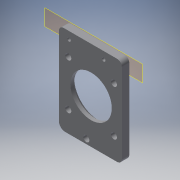
# Autodesk Inventor part: cellSTORM_inverted_chiptray_v0
Saved by Autodesk Inventor 2019.4 (Build 234330000, 330)
## iProperties
Created: 2020-11-09
Part Number: cellSTORM_inverted_chiptray_v0
Material: Generic
Document SubType Name: Modeling
Designer: diederichbenedict
Density: 1 g/cm^3
Appearance: Default
Author: diederichbenedict
Autodesk Inventor part; units mm, degrees
ref_plane "YZ Plane" through (0, 0, 0) normal (1, 0, 0) x (0, 1, 0)
ref_plane "XZ Plane" through (0, 0, 0) normal (0, 1, 0) x (-1, 0, 0)
ref_plane "XY Plane" through (0, 0, 0) normal (0, 0, 1) x (1, 0, 0)
ref_plane "Work Plane1" through (0, 0, 0) normal (0, 0, 1) x (1, 0, 0)
sketch "Sketch1" plane through (0, 0, 0) normal (0, 0, 1) x (1, 0, 0)
  line L0 (10.8382, -62.5107) -> (10.8382, 0.6668)
  line L1 (6.9805, -66.3684) -> (-18, -66.3684)
  line L2 (10.8382, -5.7047) -> (9.6808, -5.7047) construction
  line L3 (10.8382, 0.6668) -> (10.8382, 2.1422)
  line L4 (-40.1739, 0.853) -> (-40.1739, 2.1422)
  line L5 (6.9805, 6) -> (-36.3161, 6)
  circle A0 centre (-3.9646, 0) radius 1.45
  circle A1 centre (-32.0354, 0) radius 1.45
  circle A2 centre (-18, -62.5107) radius 2.45
  arc A3 (-20.665, -65.3) -> (-18, -66.3684) centre (-18, -62.5107) ccw
  arc A4 (6.9805, -66.3684) -> (10.8382, -62.5107) centre (6.9805, -62.5107) ccw
  arc A5 (-36.3161, 6) -> (-40.1739, 2.1422) centre (-36.3161, 2.1422) ccw
  arc A6 (10.8382, 2.1422) -> (6.9805, 6) centre (6.9805, 2.1422) ccw
  line L6 (-18, -66.3684) -> (-35.1739, -66.3684)
  line L7 (-40.1739, -61.3684) -> (-40.1739, 0.853)
  arc A7 (-40.1739, -61.3684) -> (-35.1739, -66.3684) centre (-35.1739, -61.3684) ccw
  point P0 (0, 0)
  point P1 (10.8382, 6)
  point P2 (-40.1739, 6)
  dimension "d6" = 2.9
  dimension "d7" = 2.9
  dimension "d32" = 90
  dimension "d46" = 5
  dimension "d47" = 62.5107
  dimension "d48" = 28.0709
  dimension "d49" = 64.067
  constraints: 16 end point, 10 point on circle, 9 tangent, 8 centre point, 5 point on line, 2 horizontal, 1 concentric, 1 equal radius, 1 perpendicular, 1 vertical
  measures "d6" diameter of A0
  measures "d7" diameter of A1
  measures "d32" angle of L1 L0
  measures "d46" radius of A7
  measures "d47" vertical distance of A3.centre A0.centre
  measures "d48" distance of A0.centre A1.centre
  measures "d49" distance of A2.centre A1.centre
extrude "Extrusion1" add sketch "Sketch1" along normal blind 6
sketch "Sketch8" plane through (0, 0, 6) normal (0, 0, 1) x (1, 0, 0)
  circle A0 centre (-18, -62.5107) radius 2.45 projected
  circle A1 centre (-32.0354, 0) radius 1.45 projected
  circle A2 centre (-3.9646, 0) radius 1.45 projected
  line L0 (-35.1739, -66.3684) -> (6.9805, -66.3684) projected
  arc A3 (6.9805, -66.3684) -> (10.8382, -62.5107) centre (6.9805, -62.5107) ccw projected
  line L1 (10.8382, -62.5107) -> (10.8382, 2.1422) projected
  arc A4 (10.8382, 2.1422) -> (6.9805, 6) centre (6.9805, 2.1422) ccw projected
  line L2 (6.9805, 6) -> (-36.3161, 6) projected
  arc A5 (-36.3161, 6) -> (-40.1739, 2.1422) centre (-36.3161, 2.1422) ccw projected
  line L3 (-40.1739, 2.1422) -> (-40.1739, -61.3684) projected
  arc A6 (-40.1739, -61.3684) -> (-35.1739, -66.3684) centre (-35.1739, -61.3684) ccw projected
  circle A7 centre (-14.0967, -30.8778) radius 16.7364
  line L4 (4.4033, -49.3778) -> (-32.5967, -49.3778)
  line L5 (-32.5967, -49.3778) -> (-32.5967, -12.3778)
  line L6 (-32.5967, -12.3778) -> (4.4033, -12.3778)
  line L7 (4.4033, -12.3778) -> (4.4033, -49.3778)
  line L8 (4.4033, -49.3778) -> (-32.5967, -12.3778) construction
  line L9 (-32.5967, -49.3778) -> (4.4033, -12.3778) construction
  circle A8 centre (-32.5967, -12.3778) radius 2.45
  circle A9 centre (4.4033, -12.3778) radius 2.45
  circle A10 centre (4.4033, -49.3778) radius 2.45
  circle A11 centre (-32.5967, -49.3778) radius 2.45
  point P0 (0, 0)
  dimension "d52" = 37
  dimension "d53" = 37
  dimension "d54" = 4.9
  dimension "d55" = 4.9
  dimension "d56" = 4.9
  dimension "d57" = 4.9
  constraints: 12 end point, 5 centre point, 4 coincident, 2 midpoint, 2 parallel, 1 horizontal, 1 perpendicular
  measures "d52" distance of L5.end L6.end
  measures "d53" distance of L4.end L5.end
  measures "d54" diameter of A8
  measures "d55" diameter of A9
  measures "d56" diameter of A10
  measures "d57" diameter of A11
extrude "Extrusion7" cut sketch "Sketch8" against normal through all contours A7 | A11 L5 L4 | L4 L5 A11 | A10 L7 L4 | L4 L7 A10 | A8 L6 L5 | L5 L6 A8 | A9 L6 L7 | L7 L6 A9
chamfer "Chamfer3" distance 3 angle 45 1 edges at (-30.8332, -30.8778, 0)
body "Solid1"
